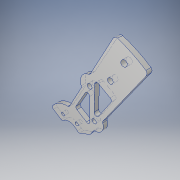
# Autodesk Inventor part: Doubler
Saved by Autodesk Inventor 2019 (Build 230136000, 136)
## iProperties
Created: 2019-01-25
Part Number: Doubler
Material: Aluminum 6061
Document SubType Name: Modeling
Designer: Adhik
Density: 2.7 g/cm^3
Appearance: Aluminum - Flat
Author: Adhik
Autodesk Inventor part; units mm, degrees
ref_plane "YZ Plane" through (0, 0, 0) normal (1, 0, 0) x (0, 1, 0)
ref_plane "XZ Plane" through (0, 0, 0) normal (0, 1, 0) x (-1, 0, 0)
ref_plane "XY Plane" through (0, 0, 0) normal (0, 0, 1) x (1, 0, 0)
sketch "Sketch1" plane through (0, 0, 0) normal (0, 0, 1) x (1, 0, 0)
  circle A0 centre (11.9062, -20.6222) radius 2.5908 construction
  circle A1 centre (-23.8125, 0) radius 2.5908 construction
  circle A2 centre (11.9063, 20.6222) radius 2.5908 projected
  circle A3 centre (23.8125, 0) radius 2.5908 construction
  circle A4 centre (-11.9062, 20.6222) radius 2.5908 projected
  circle A5 centre (-11.9062, -20.6222) radius 2.5908 construction
  circle A6 centre (0, 0) radius 14.478 construction
  circle A7 centre (57.15, 98.9867) radius 3.175 projected
  circle A8 centre (69.85, 120.9837) radius 3.175 projected
  circle A9 centre (98.9867, 57.15) radius 3.175 construction
  circle A10 centre (120.9837, 69.85) radius 3.175 construction
  circle A11 centre (114.3, 0) radius 3.175 construction
  circle A12 centre (139.7, 0) radius 3.175 construction
  circle A13 centre (98.9867, -57.15) radius 3.175 construction
  circle A14 centre (120.9837, -69.85) radius 3.175 construction
  circle A15 centre (57.15, -98.9867) radius 3.175 construction
  circle A16 centre (69.85, -120.9837) radius 3.175 construction
  circle A17 centre (0, -114.3) radius 3.175 construction
  circle A18 centre (0, -139.7) radius 3.175 construction
  circle A19 centre (-57.15, -98.9867) radius 3.175 construction
  circle A20 centre (-69.85, -120.9837) radius 3.175 construction
  circle A21 centre (-98.9867, -57.15) radius 3.175 construction
  circle A22 centre (-120.9837, -69.85) radius 3.175 construction
  circle A23 centre (-114.3, 0) radius 3.175 construction
  circle A24 centre (-139.7, 0) radius 3.175 construction
  circle A25 centre (-98.9867, 57.15) radius 3.175 construction
  circle A26 centre (-120.9837, 69.85) radius 3.175 construction
  circle A27 centre (-57.15, 98.9867) radius 3.175 construction
  circle A28 centre (-69.85, 120.9837) radius 3.175 construction
  circle A29 centre (0, 114.3) radius 3.175 construction
  circle A30 centre (0, 139.7) radius 3.175 construction
  circle A31 centre (0, 0) radius 152.4 construction
  arc A32 (92.1001, 121.4221) -> (59.1046, 140.4721) centre (0, 0) ccw
  line L0 (59.1046, 140.4721) -> (0, 38.1)
  line L1 (92.1001, 121.4221) -> (32.9956, 19.05)
  line L2 (69.85, 120.9837) -> (0, 0) construction
  line L3 (0, 0) -> (-12.5383, 7.239) construction
  line L4 (0, -263.7526) -> (0, 221.7588) construction
  arc A33 (0, 38.1) -> (-32.9956, 19.05) centre (0, 0) ccw
  line L5 (12.5383, 7.239) -> (0, 0) construction
  arc A34 (13.9131, 8.0328) -> (-13.9131, 8.0328) centre (0, 0) ccw
  line L6 (-13.9131, 8.0328) -> (-32.9956, 19.05)
  line L7 (32.9956, 19.05) -> (13.9131, 8.0328)
  dimension "d1" = 38.1
  dimension "d19" = 1.5875
  constraints: 16 end point, 8 point on circle, 3 centre point, 2 coincident, 2 collinear, 2 concentric, 2 parallel, 1 point on line, 1 vertical, 4 other
  measures "d1" distance between parallel lines of L1 L0
  measures "d19" radial gap between concentric circles of A34 A6
extrude "Extrusion1" add sketch "Sketch1" along normal blind 6.35
sketch "Sketch2" plane through (0, 0, 6.35) normal (0, 0, 1) x (1, 0, 0)
  line L0 (12.0202, 46.2196) -> (26.5051, 71.3083)
  line L1 (32.4298, 69.7208) -> (32.4298, 36.2693)
  line L2 (27.6673, 33.5196) -> (13.1824, 41.8825)
  line L3 (59.1046, 140.4721) -> (0, 38.1) construction
  arc A0 (0, 38.1) -> (-32.9956, 19.05) centre (0, 0) ccw construction
  line L4 (38.7798, 87.0693) -> (38.7798, 53.6178)
  line L5 (43.5423, 89.8189) -> (58.0272, 81.456)
  line L6 (59.1893, 77.1189) -> (44.7044, 52.0303)
  line L7 (32.9956, 19.05) -> (92.1001, 121.4221) construction
  circle A1 centre (11.9063, 20.6222) radius 2.5908 construction
  arc A2 (12.0202, 46.2196) -> (13.1824, 41.8825) centre (14.7699, 44.6321) ccw
  arc A3 (32.4298, 69.7208) -> (26.5051, 71.3083) centre (29.2548, 69.7208) ccw
  arc A4 (27.6673, 33.5196) -> (32.4298, 36.2693) centre (29.2548, 36.2693) ccw
  arc A5 (38.7798, 53.6178) -> (44.7044, 52.0303) centre (41.9548, 53.6178) ccw
  arc A6 (43.5423, 89.8189) -> (38.7798, 87.0693) centre (41.9548, 87.0693) ccw
  arc A7 (59.1893, 77.1189) -> (58.0272, 81.456) centre (56.4397, 78.7064) ccw
  point P0 (0, 0)
  point P1 (32.4298, 30.77)
  point P2 (38.7798, 92.5685)
  dimension "d4" = 6.35
  dimension "d5" = 6.35
  dimension "d6" = 6.35
  dimension "d7" = 19.05
  dimension "d8" = 3.175
  constraints: 12 end point, 12 point on circle, 12 tangent, 6 centre point, 6 point on line, 5 equal radius, 2 parallel, 2 perpendicular, 1 vertical
  measures "d4" distance between parallel lines of L3 L0
  measures "d5" distance between parallel lines of L7 L6
  measures "d6" distance between parallel lines of L1 L4
  measures "d7" distance from line of A1.centre L2
  measures "d8" radius of A2
extrude "Extrusion2" cut sketch "Sketch2" against normal blind 6.35
sketch "Sketch3" plane through (0, 0, 6.35) normal (0, 0, 1) x (1, 0, 0)
  circle A0 centre (32.4298, 81.57) radius 3.175
  line L0 (12.0202, 46.2196) -> (26.5051, 71.3083) construction
  circle A1 centre (38.7798, 41.7685) radius 3.175
  line L1 (59.1893, 77.1189) -> (44.7044, 52.0303) construction
  line L2 (32.4298, 69.7208) -> (32.4298, 36.2693) construction
  line L3 (38.7798, 53.6178) -> (38.7798, 87.0693) construction
  point P0 (0, 0)
  dimension "d12" = 6.35
  constraints: 4 point on line, 2 centre point, 1 equal radius
  measures "d12" diameter of A0
extrude "Extrusion3" cut sketch "Sketch3" against normal through all
sketch "Sketch4" plane through (0, 0, 6.35) normal (0, 0, 1) x (1, 0, 0)
  arc A0 (32.4298, 94.27) -> (21.4313, 75.22) centre (32.4298, 81.57) ccw
  circle A1 centre (32.4298, 81.57) radius 3.175 construction
  line L0 (32.4298, 94.27) -> (21.4313, 75.22)
  line L1 (59.1046, 140.4721) -> (0, 38.1) construction
  arc A2 (38.7798, 29.0685) -> (49.7783, 48.1185) centre (38.7798, 41.7685) ccw
  line L2 (49.7783, 48.1185) -> (38.7798, 29.0685)
  circle A3 centre (38.7798, 41.7685) radius 3.175 construction
  line L3 (32.9956, 19.05) -> (92.1001, 121.4221) construction
  point P0 (0, 0)
  point P1 (57.6913, 138.0243)
  point P2 (0.8924, 39.6457)
  point P3 (33.4209, 19.7868)
  point P4 (90.6869, 118.9743)
  dimension "d15" = 12.7
  constraints: 4 end point, 4 point on circle, 2 centre point, 2 coincident, 2 collinear, 1 parallel
  measures "d15" radius of A0
extrude "Extrusion4" add sketch "Sketch4" against normal blind 6.35
fillet "Fillet2" radius 3.175 11 edges at (-32.9956, 19.05, 3.175) (0, 38.1, 3.175) (32.4298, 94.27, 3.175) (21.4313, 75.22, 3.175) (59.1046, 140.4721, 3.175) (92.1001, 121.4221, 3.175) (49.7783, 48.1185, 3.175) (38.7798, 29.0685, 3.175) (32.9956, 19.05, 3.175) (-13.9131, 8.0328, 3.175) (13.9131, 8.0328, 3.175)
equation "\"d5\" = d4"
equation "\"d6\" = d4"
body "Solid1"
